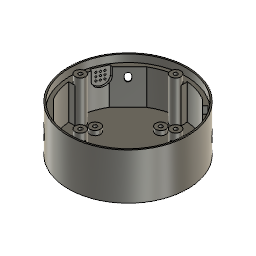
LAMP - BASE (Autodesk Fusion 360 design; units mm, degrees)
part number: 2026-05-21-10-57-22-259
Autodesk Fusion 360 part; units mm, degrees
note: some values were not read from the file. Set by a fixed rule: which sketch regions a step uses.
sketch "Sketch1" plane through (0, 0, 0) normal (0, 0, 1) x (1, 0, 0)
  circle A0 centre (0, 0) radius 40
  circle A1 centre (0, 0) radius 39
  dimension "d1" = 80
  dimension "d2" = 78
  constraint coincident A0.centre A1.centre
  measures "d1" diameter of A0
  measures "d2" diameter of A1
extrude "Extrude1" add sketch "Sketch1" along normal blind 31
sketch "Sketch2" plane through (0, 0, 0) normal (0, 0, 1) x (1, 0, 0)
  circle A0 centre (0, 0) radius 39
  circle A1 centre (0, 0) radius 36.5
  dimension "d5" = 78
  dimension "d6" = 73
  constraint coincident A0.centre A1.centre
  constraint concentric A0 A1
  measures "d5" diameter of A0
  measures "d6" diameter of A1
extrude "Extrude2" add sketch "Sketch2" along normal blind 2.5 contours A0 | A1
extrude "Extrude3" add sketch "Sketch2" along normal blind 26
sketch "Sketch3" plane through (0, 0, 2.5) normal (0, 0, 1) x (-1, 0, 0)
  circle A0 centre (0, 0) radius 36.5
  circle A1 centre (0, 22) radius 3.5
  circle A2 centre (0, 22) radius 1.25
  circle A3 centre (-22, 0) radius 3.5
  circle A4 centre (-22, 0) radius 1.25
  circle A5 centre (0, -22) radius 3.5
  circle A6 centre (0, -22) radius 1.25
  circle A7 centre (22, 0) radius 3.5
  circle A8 centre (22, 0) radius 1.25
  dimension "d11" = 7
  dimension "d12" = 2.5
  dimension "d13" = 22
  dimension "d15" = 360
  constraint concentric A1 A2
  constraint vertical A0.centre A1.centre
  measures "d11" diameter of A1
  measures "d12" diameter of A2
  measures "d13" distance of A0.centre A1.centre
extrude "Extrude4" add sketch "Sketch3" along normal blind 3 contours A1 | A3 | A5 | A7
sketch "Sketch4" plane through (0, 0, 2.5) normal (0, 0, 1) x (-1, 0, 0)
  circle A0 centre (0, -22) radius 3.5
  circle A1 centre (-22, 0) radius 3.5
  circle A2 centre (0, 0) radius 36.5
  circle A3 centre (22, 0) radius 3.5
  circle A4 centre (0, 22) radius 3.5
  circle A5 centre (0, 32) radius 3.5
  circle A6 centre (0, 32) radius 1.25
  circle A7 centre (0, 0) radius 36.5
  line L0 (-3.5, 32) -> (-3.5, 36.3318)
  line L1 (3.5, 32) -> (3.5, 36.3318)
  dimension "d18" = 7
  dimension "d19" = 2.5
  dimension "d20" = 32
  constraint concentric A5 A6
  constraint vertical A2.centre A5.centre
  constraint coincident A5 L0.start
  constraint coincident A2 L0.end
  constraint tangent A5 L0
  constraint vertical L0
  constraint coincident A5 L1.start
  constraint coincident A2 L1.end
  constraint tangent A5 L1
  constraint parallel L0 L1
  measures "d18" diameter of A5
  measures "d19" diameter of A6
  measures "d20" vertical distance of A2.centre A5.centre
extrude "Extrude5" add sketch "Sketch4" along normal blind 28.5 contours A5
extrude "Extrude6" add sketch "Sketch4" along normal blind 23.5 contours A2 A5 A7 L0 L1 picked at (-2.1394, 35.9481)
pattern_circular "C-Pattern1" count 4 over 360 about axis through (0, 0, 1.75) along (0, 0, 1) of "Extrude5", "Extrude6"
sketch "Sketch5" plane through (0, 0, 26) normal (0, 0, 1) x (-1, 0, 0)
  arc A0 (36.3318, 3.5) -> (3.5, 36.3318) centre (0, 0) ccw
  circle A1 centre (0, 0) radius 39
  arc A2 (3.5, -36.3318) -> (36.3318, -3.5) centre (0, 0) ccw
  arc A3 (-36.3318, -3.5) -> (-3.5, -36.3318) centre (0, 0) ccw
  arc A4 (-3.5, 36.3318) -> (-36.3318, 3.5) centre (0, 0) ccw
  arc A5 (36.3318, 3.5) -> (3.5, 36.3318) centre (0, 0) ccw
  line L0 (31.3167, -18.7487) -> (18.7432, -31.32)
  line L1 (0, 0) -> (0, -13.7257) construction
  line L2 (0, 0) -> (13.0082, 0) construction
  line L3 (-31.3167, -18.7487) -> (-18.7432, -31.32)
  line L4 (31.3167, 18.7487) -> (18.7432, 31.32)
  line L5 (36.3318, 3.5) -> (32, 3.5)
  arc A6 (32, -3.5) -> (32, 3.5) centre (32, 0) ccw
  line L6 (32, -3.5) -> (36.3318, -3.5)
  arc A7 (3.5, -36.3318) -> (36.3318, -3.5) centre (0, 0) ccw
  line L7 (3.5, -36.3318) -> (3.5, -32)
  arc A8 (-3.5, -32) -> (3.5, -32) centre (0, -32) ccw
  line L8 (-3.5, -32) -> (-3.5, -36.3318)
  arc A9 (-36.3318, -3.5) -> (-3.5, -36.3318) centre (0, 0) ccw
  line L9 (-36.3318, -3.5) -> (-32, -3.5)
  arc A10 (-32, 3.5) -> (-32, -3.5) centre (-32, 0) ccw
  line L10 (-32, 3.5) -> (-36.3318, 3.5)
  arc A11 (-3.5, 36.3318) -> (-36.3318, 3.5) centre (0, 0) ccw
  line L11 (-3.5, 36.3318) -> (-3.5, 32)
  arc A12 (3.5, 32) -> (-3.5, 32) centre (0, 32) ccw
  line L12 (3.5, 32) -> (3.5, 36.3318)
  dimension "d27" = 17.78
  dimension "d28" = 16.046
  constraint coincident A0.centre A1.centre
  constraint vertical L1
  constraint perpendicular L1 L2
  constraint symmetric L0.start L1 L3.start
  constraint symmetric L0.end L1 L3.end
  constraint symmetric L0.start L2 L4.start
  constraint symmetric L0.end L2 L4.end
  measures "d27" distance of L0.start L0.end
  measures "d28" distance of A2.start L0.end
extrude "Extrude7" add sketch "Sketch5" against normal blind 23.5 contours A0 A5 L4 | A2 L0 A7 | A3 L3 A9
sketch "Sketch6" plane through (-25.03, -25.0344, 0) normal (0.707045, 0.707169, 0) x (-0.707169, 0.707045, 0)
  line L0 (-8.89, 2.5) -> (8.89, 2.5)
  line L1 (8.89, 2.5) -> (8.89, 26)
  line L2 (8.89, 26) -> (-8.89, 26)
  line L3 (-8.89, 26) -> (-8.89, 2.5)
  circle A0 centre (0, 13.5) radius 4.5
  dimension "d31" = 9
  dimension "d32" = 13.5
  constraint vertical origin A0.centre
  measures "d31" diameter of A0
  measures "d32" distance of origin A0.centre
extrude "Extrude8" cut sketch "Sketch6" against normal through all contours A0
sketch "Sketch7" plane through (-25.03, 25.0344, 0) normal (0.707045, -0.707169, 0) x (0.707169, 0.707045, 0)
  line L0 (-8.89, 2.5) -> (8.89, 2.5)
  line L1 (8.89, 2.5) -> (8.89, 26)
  line L2 (8.89, 26) -> (-8.89, 26)
  line L3 (-8.89, 26) -> (-8.89, 2.5)
  line L4 (-1.725, 21.025) -> (-1.725, 18.975)
  arc A0 (-1.725, 18.975) -> (1.725, 18.975) centre (0, 18.975) ccw
  line L5 (1.725, 18.975) -> (1.725, 21.025)
  arc A1 (1.725, 21.025) -> (-1.725, 21.025) centre (0, 21.025) ccw
  line L6 (0, 22.75) -> (0, 17.25) construction
  dimension "d34" = 3.45
  dimension "d35" = 5.5
  dimension "d36" = 14.75
  constraint tangent L4 A0
  constraint tangent A0 L5
  constraint parallel L4 L5
  constraint tangent L5 A1
  constraint tangent L4 A1
  constraint coincident A1 L6.start
  constraint coincident A0 L6.end
  constraint coincident A0.centre L6
  constraint coincident A1.centre L6
  constraint vertical L6
  constraint vertical origin A0.centre
  measures "d34" distance of L4 L5
  measures "d35" distance of L6.start L6.end
  measures "d36" distance of L0 L6.end
extrude "Extrude9" cut sketch "Sketch7" against normal blind 0.698 contours L4 A0 L5 A1
extrude "Extrude10" cut sketch "Sketch7" against normal through all draft 37 from surface at -0.698 contours L4 A0 L5 A1
sketch "Sketch8" plane through (25.03, 25.0344, 0) normal (-0.707045, -0.707169, 0) x (0.707169, -0.707045, 0)
  line L0 (8.89, 26) -> (-8.89, 26)
  line L1 (-8.89, 26) -> (-8.89, 2.5)
  line L2 (-8.89, 2.5) -> (8.89, 2.5)
  line L3 (8.89, 2.5) -> (8.89, 26)
  circle A0 centre (0, 11) radius 3.5
  line L4 (-3.5, 26) -> (-3.5, 11)
  line L5 (3.5, 26) -> (3.5, 11)
  dimension "d41" = 7
  dimension "d42" = 11
  constraint vertical origin A0.centre
  constraint coincident L0 L4.start
  constraint perpendicular L0 L4
  constraint coincident L0 L5.start
  constraint coincident A0 L5.end
  constraint coincident A0 L4.end
  constraint tangent A0 L4
  constraint tangent A0 L5
  constraint vertical L5
  measures "d41" diameter of A0
  measures "d42" vertical distance of origin A0.centre
extrude "Extrude11" cut sketch "Sketch8" against normal blind 2.6 contours L0 A0 L4 L5 | A0
extrude "Extrude12" cut sketch "Sketch8" against normal blind 4.6 contours A0
sketch "Sketch9" plane through (0, 0, 26) normal (0, 0, 1) x (-1, 0, 0)
  circle A0 centre (0, 0) radius 39
  line L0 (-22.5549, -27.509) -> (-24.3932, -29.3477)
  line L1 (-24.3932, -29.3477) -> (-29.3434, -24.3983)
  line L2 (-29.3434, -24.3983) -> (-27.505, -22.5597)
  line L3 (-27.505, -22.5597) -> (-31.3167, -18.7487)
  arc A1 (-36.3318, -3.5) -> (-31.3167, -18.7487) centre (0, 0) ccw
  line L4 (-36.3318, -3.5) -> (-32, -3.5)
  arc A2 (-32, 3.5) -> (-32, -3.5) centre (-32, 0) ccw
  line L5 (-32, 3.5) -> (-36.3318, 3.5)
  arc A3 (-3.5, 36.3318) -> (-36.3318, 3.5) centre (0, 0) ccw
  line L6 (-3.5, 36.3318) -> (-3.5, 32)
  arc A4 (3.5, 32) -> (-3.5, 32) centre (0, 32) ccw
  line L7 (3.5, 32) -> (3.5, 36.3318)
  arc A5 (18.7432, 31.32) -> (3.5, 36.3318) centre (0, 0) ccw
  line L8 (18.7432, 31.32) -> (31.3167, 18.7487)
  arc A6 (36.3318, 3.5) -> (31.3167, 18.7487) centre (0, 0) ccw
  line L9 (36.3318, 3.5) -> (32, 3.5)
  arc A7 (32, -3.5) -> (32, 3.5) centre (32, 0) ccw
  line L10 (32, -3.5) -> (36.3318, -3.5)
  arc A8 (31.3167, -18.7487) -> (36.3318, -3.5) centre (0, 0) ccw
  line L11 (31.3167, -18.7487) -> (18.7432, -31.32)
  arc A9 (3.5, -36.3318) -> (18.7432, -31.32) centre (0, 0) ccw
  line L12 (3.5, -36.3318) -> (3.5, -32)
  arc A10 (-3.5, -32) -> (3.5, -32) centre (0, -32) ccw
  line L13 (-3.5, -32) -> (-3.5, -36.3318)
  arc A11 (-18.7432, -31.32) -> (-3.5, -36.3318) centre (0, 0) ccw
  line L14 (-18.7432, -31.32) -> (-22.5549, -27.509)
  line L15 (31.3167, -18.7487) -> (18.7432, -31.32)
  arc A12 (31.3167, -18.7487) -> (36.3318, -3.5) centre (0, 0) ccw
  arc A13 (3.5, -36.3318) -> (18.7432, -31.32) centre (0, 0) ccw
  line L16 (36.4457, -10.9357) -> (32.1385, -20.5117)
  line L17 (32.1385, -20.5117) -> (30.3555, -19.7097)
  line L18 (36.4457, -10.9357) -> (35.0184, -10.2938)
  dimension "d50" = 10.5
  dimension "d51" = 17.212
  dimension "d52" = 1.565
  dimension "d53" = 1.955
  constraint coincident L15 L17.end
  constraint perpendicular L16 L17
  constraint coincident A8 L18.end
  constraint perpendicular L16 L18
  measures "d50" distance of L16.start L16.end
  measures "d51" distance of L11.end L16.end
  measures "d52" distance of L16.start L18.end
  measures "d53" distance of L16.end L17.end
extrude "Extrude13" cut sketch "Sketch9" against normal blind 5.8 contours A8 L11 L15 A12 L16 L17 L18
ref_plane "WorkPlane1" through (-30.3555, 19.7097, 26) normal (0.938263, -0.345923, 0) x (0.345923, 0.938263, 0)
sketch "Sketch10" plane through (-33.1202, 12.2109, 0) normal (0.938263, -0.345923, 0) x (0.345923, 0.938263, 0)
  line L0 (-2.4554, 20.2) -> (-2.4554, 26)
  line L1 (6.7581, 20.2) -> (-2.4554, 20.2)
  line L2 (7.9922, 20.2) -> (6.7581, 20.2)
  line L3 (7.9922, 26) -> (7.9922, 20.2)
  arc A0 (-2.4554, 20.2) -> (7.9922, 20.2) centre (2.7684, 20.2) ccw
  constraint tangent L3 A0
extrude "Extrude14" cut sketch "Sketch10" along normal up to surface end surface through (-36.4457, 10.9357, 26) normal (0.911992, -0.410207, 0) offset 0
sketch "Sketch11" plane through (-34.4041, 15.4747, 0) normal (0.911992, -0.410207, 0) x (0.410207, 0.911992, 0)
  line L0 (5.523, 26) -> (-4.977, 26)
  line L1 (-4.977, 26) -> (-4.977, 20.2)
  line L2 (-4.977, 20.2) -> (-5.0858, 20.2)
  ellipse E0 centre (0.1506, 20.2) end of major axis (-5.0858, 20.2) minor radius 5.2238 (-5.0858, 20.2) -> (5.387, 20.2) ccw
  line L3 (5.387, 20.2) -> (5.523, 20.2)
  line L4 (5.523, 20.2) -> (5.523, 26)
  circle A0 centre (2.622, 23.4) radius 0.6
  circle A1 centre (0.304, 23.4) radius 0.6
  circle A2 centre (-2.014, 23.4) radius 0.6
  circle A3 centre (2.622, 20.9) radius 0.6
  circle A4 centre (0.304, 20.9) radius 0.6
  circle A5 centre (-2.014, 20.9) radius 0.6
  circle A6 centre (2.622, 18.4) radius 0.6
  circle A7 centre (0.304, 18.4) radius 0.6
  circle A8 centre (-2.014, 18.4) radius 0.6
  dimension "d59" = 1.2
  dimension "d60" = 2.6
  dimension "d61" = 2.901
  dimension "d62" = 1.2
  dimension "d63" = 1.2
  dimension "d64" = 2.318
  dimension "d65" = 2.318
  dimension "d68" = 0
  dimension "d69" = -5
  constraint horizontal A0.centre A1.centre
  constraint horizontal A1.centre A2.centre
  measures "d59" diameter of A0
  measures "d60" distance of L0 A0.centre
  measures "d61" distance of L4 A0.centre
  measures "d62" diameter of A1
  measures "d63" diameter of A2
  measures "d64" distance of A0.centre A1.centre
  measures "d65" distance of A1.centre A2.centre
extrude "Extrude15" cut sketch "Sketch11" against normal through all contours A0 | A1 | A2 | A3 | A4 | A5 | A6 | A7 | A8
equation "d9 = 23.5 mm + 2.5 mm"
